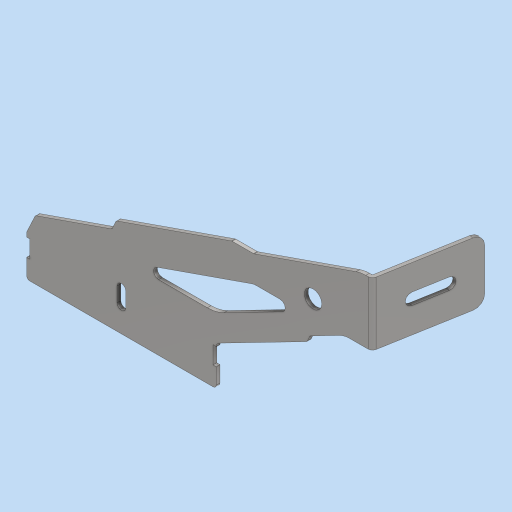
# Autodesk Inventor part: 0 零件
Saved by Autodesk Inventor 2023 (Build 270158000, 158)
## iProperties
Created: 2020-11-03
Part Number: 0 零件
Material: 不鏽鋼
Document SubType Name: Sheet Metal
Designer: p2013
Density: 8 g/cm^3
Appearance: SUS-2B
Sheet Metal Rule: 預設 mm (_M)
Flat Pattern Width: 8.37536 cm
Flat Pattern Length: 32.0542 cm
Flat Pattern Area: 268.466 cm^2
Sheet Metal Width: 83.754 mm
Sheet Metal Length: 320.542 mm
Sheet Metal Area: 26846.580 mm^2
Author: p2013
Autodesk Inventor part; units mm, degrees
ref_plane "YZ Plane" through (0, 0, 0) normal (1, 0, 0) x (0, 1, 0)
ref_plane "XZ Plane" through (0, 0, 0) normal (0, 1, 0) x (-1, 0, 0)
ref_plane "XY Plane" through (0, 0, 0) normal (0, 0, 1) x (1, 0, 0)
sketch "草圖1" plane through (0, 0, 0) normal (0, 0, 1) x (1, 0, 0)
  line L0 (0, 0) -> (-7.8042, 0) construction
  line L1 (0, 0) -> (0, -16.694) construction
  line L2 (0, 2) -> (0, 13)
  line L3 (234.1969, 118.5697) -> (234.1969, 75.5697)
  line L4 (130, 19.7875) -> (130, 13) construction
  line L5 (128, 0) -> (2, 0)
  line L6 (234.1969, 118.5697) -> (292.1969, 118.5697)
  line L7 (299.1969, 111.5697) -> (299.1969, 82.5697)
  line L8 (292.1969, 75.5697) -> (234.1969, 75.5697)
  line L9 (256.1969, 101.0697) -> (278.1969, 101.0697)
  arc A0 (278.1969, 93.0697) -> (278.1969, 101.0697) centre (278.1969, 97.0697) ccw
  line L10 (278.1969, 93.0697) -> (256.1969, 93.0697)
  arc A1 (256.1969, 101.0697) -> (256.1969, 93.0697) centre (256.1969, 97.0697) ccw
  line L11 (65, 14) -> (65, 14) construction
  line L12 (6.5315, 40.9329) -> (57.8672, 58.8322)
  line L13 (232.5836, 118.5697) -> (234.1969, 118.5697)
  line L14 (234.1969, 75.5697) -> (221.4643, 75.5697)
  line L15 (214.6027, 73.9083) -> (194.8909, 63.7682)
  arc A2 (299.1969, 111.5697) -> (292.1969, 118.5697) centre (292.1969, 111.5697) ccw
  arc A3 (292.1969, 75.5697) -> (299.1969, 82.5697) centre (292.1969, 82.5697) ccw
  line L16 (0, 25) -> (2.15, 25)
  line L17 (2.15, 25) -> (2.15, 13)
  line L18 (2.15, 13) -> (0, 13)
  line L19 (0, 13) -> (0, 25) construction
  line L20 (65, 0) -> (65, 27) construction
  line L21 (130, 25) -> (127.85, 25)
  line L22 (127.85, 25) -> (127.85, 13)
  line L23 (127.85, 13) -> (130, 13)
  line L24 (130, 13) -> (130, 19.7875) construction
  arc A4 (0, 2) -> (2, 0) centre (2, 2) ccw
  arc A5 (128, 0) -> (130, 2) centre (128, 2) ccw
  line L25 (0, 13) -> (0, 25) construction
  line L26 (0, 25) -> (0, 27.6675)
  line L27 (130, 19.7875) -> (130, 25) construction
  line L28 (130, 13) -> (130, 2)
  line L29 (123.9345, 45) -> (90.5004, 45)
  line L30 (157.566, 75) -> (173.8509, 75)
  line L31 (89.3481, 51.8049) -> (154.2737, 74.4425)
  line L32 (175.452, 68.3877) -> (135.3705, 47.769)
  arc A6 (175.452, 68.3877) -> (173.8509, 75) centre (173.8509, 71.5) ccw
  arc A7 (89.3481, 51.8049) -> (90.5004, 45) centre (90.5004, 48.5) ccw
  arc A8 (123.9345, 45) -> (135.3705, 47.769) centre (123.9345, 70) ccw
  arc A9 (157.566, 75) -> (154.2737, 74.4425) centre (157.566, 65) ccw
  line L33 (219.0826, 147.5779) -> (251.7371, 53.9233) construction
  arc A10 (232.5836, 118.5697) -> (225.9989, 117.4547) centre (232.5836, 98.5697) ccw
  arc A11 (221.4643, 75.5697) -> (214.6027, 73.9083) centre (221.4643, 60.5697) ccw
  line L34 (5.6659, 40.1505) -> (0.1405, 28.3014)
  line L35 (58.7328, 59.6146) -> (61.1461, 64.79)
  line L36 (62.0118, 65.5724) -> (140.4352, 92.9164)
  line L37 (140.9291, 93) -> (155.6079, 93)
  line L38 (131.899, 27.9903) -> (191.8622, 58.8365)
  line L39 (192.6867, 59.7276) -> (193.9617, 62.764)
  line L40 (194.2436, 63.4352) -> (119.2993, 24.8824) construction
  line L41 (156.1018, 93.0836) -> (225.9989, 117.4547)
  line L42 (58.4652, 59.0406) -> (155.8619, 93) construction
  arc A12 (194.8909, 63.7682) -> (193.9617, 62.764) centre (195.8058, 61.9897) ccw
  arc A13 (57.8672, 58.8322) -> (58.7328, 59.6146) centre (57.3734, 60.2485) ccw
  arc A14 (155.6079, 93) -> (156.1018, 93.0836) centre (155.6079, 94.5) ccw
  arc A15 (140.9291, 93) -> (140.4352, 92.9164) centre (140.9291, 91.5) ccw
  arc A16 (62.0118, 65.5724) -> (61.1461, 64.79) centre (62.5056, 64.1561) ccw
  arc A17 (191.8622, 58.8365) -> (192.6867, 59.7276) centre (191.0504, 60.4147) ccw
  circle A18 centre (196.4588, 86.5036) radius 6
  line L43 (130, 25) -> (130, 24.8779)
  arc A19 (131.899, 27.9903) -> (130, 24.8779) centre (133.5, 24.8779) ccw
  arc A20 (6.5315, 40.9329) -> (5.6659, 40.1505) centre (7.0253, 39.5165) ccw
  arc A21 (0.1405, 28.3014) -> (0, 27.6675) centre (1.5, 27.6675) ccw
  arc A22 (65, 24) -> (68, 27) centre (65, 27) ccw construction
  line L44 (62, 27) -> (62, 17)
  arc A23 (62, 17) -> (68, 17) centre (65, 17) ccw
  line L45 (68, 17) -> (68, 27)
  arc A24 (62, 27) -> (65, 24) centre (65, 27) ccw construction
  arc A25 (68, 27) -> (62, 27) centre (65, 27) ccw
  point P0 (130, 0)
  point P1 (299.1969, 118.5697)
  point P2 (299.1969, 75.5697)
  point P3 (0, 28)
  point P4 (130, 30.3871)
  point P5 (5.9335, 40.7244)
  point P6 (229.1969, 118.5697)
  point P7 (0, 10.2)
  point P8 (130, 28)
  point P9 (130, 10.2)
  point P10 (61.4138, 65.364)
  point P11 (140.6751, 93)
  point P12 (192.4366, 59.132)
  dimension "d0" = 130
  dimension "d2" = 43
  dimension "d3" = 65
  dimension "d4" = 8
  dimension "d5" = 30
  dimension "d7" = 18
  dimension "d14" = 14
  dimension "d17" = 21.5
  dimension "d21" = 28
  dimension "d23" = 5
  dimension "d24" = 7
  dimension "d33" = 8
  dimension "d39" = 12
  dimension "d41" = 13
  dimension "d42" = 2
  dimension "d46" = 17
  dimension "d47" = 13
  dimension "d49" = 3.5
  dimension "d50" = 3.5
  dimension "d51" = 25
  dimension "d52" = 10
  dimension "d57" = 4.7213
  dimension "d58" = 132.7034
  dimension "d60" = 19.222
  dimension "d61" = 20
  dimension "d62" = 15
  dimension "d65" = 118.5697
  dimension "d66" = 65
  dimension "d67" = 5
  dimension "d69" = 65
  dimension "d70" = 3
  dimension "d72" = 2
  dimension "d73" = 1.5
  dimension "d76" = 18
  dimension "d77" = 12
  dimension "d79" = 40
  dimension "d80" = 3.5
  dimension "d81" = 13.5
  dimension "d82" = 13.5
  dimension "d83" = 75
  dimension "d84" = 27.9903
  dimension "d85" = 45
  dimension "d86" = 55
  dimension "d87" = 1.5
  dimension "d91" = 10
  dimension "d93" = 6
  dimension "d94" = 17
  dimension "d95" = 125.7
  constraints: 94 end point, 54 tangent, 50 point on circle, 33 point on line, 26 centre point, 23 parallel, 9 horizontal, 8 perpendicular, 7 vertical, 6 equal radius, 5 symmetric about line, 3 vertical alignment, 2 coincident, 2 midpoint
  measures "d0" distance between parallel lines of L4 L2
  measures "d2" distance between parallel lines of L6 L8
  measures "d3" distance between parallel lines of L7 L3
  measures "d4" distance between parallel lines of L10 L9
  measures "d7" distance edge to line of A1 L3
  measures "d14" distance from line of L5 L11.start
  measures "d17" distance from line of L6 A0.centre
  measures "d21" distance of L0.start point (0, 28)
  measures "d23" distance of point (229.197, 118.57) L3.start
  measures "d24" radius of A2
  measures "d33" angle of L15 L12
  measures "d39" distance between parallel lines of L18 L16
  measures "d41" distance between parallel lines of L18 L5
  measures "d42" radius of A4
  measures "d46" distance between parallel lines of L12 L31
  measures "d47" distance between parallel lines of L15 L32
  measures "d49" radius of A6
  measures "d50" radius of A7
  measures "d51" radius of A8
  measures "d52" radius of A9
  measures "d57" distance from line of L3.start L33
  measures "d58" distance from line of point (130, 0) L33
  measures "d60" angle of L5 L12
  measures "d61" radius of A10
  measures "d62" radius of A11
  measures "d65" distance between parallel lines of L5 L6
  measures "d66" angle of L5 L34
  measures "d67" distance between parallel lines of L36 L12
  measures "d69" angle of L5 L35
  measures "d70" distance between parallel lines of L15 L38
  measures "d72" radius of A12
  measures "d73" radius of A13
  measures "d76" distance between parallel lines of L37 L30
  measures "d77" diameter of A18
  measures "d79" angle of L38 L39
  measures "d80" radius of A19
  measures "d81" distance edge to line of A18 L15
  measures "d82" distance edge to line of A18 L41
  measures "d83" distance between parallel lines of L5 L30
  measures "d84" distance from line of L38.start L5
  measures "d85" distance between parallel lines of L5 L29
  measures "d86" distance of point (5.933, 40.724) L12.end
  measures "d87" radius of A20
  measures "d91" distance of L20.end A23.centre
  measures "d93" distance between parallel lines of L45 L44
  measures "d94" distance from line of L5 A23.centre
  measures "d95" distance between parallel lines of L17 L22
extrude "擠出1" add sketch "草圖1" along normal blind 2.5
bend part "折彎零件1" radius 0.5 angle 80 line through (234.1969, 118.5697, 0) along (0, -1, 0) centre toward (0, 0, -1) moving side (1, 0, 0) both sides no
ref_plane "工作平面1" through (65, 2, 0) normal (-1, 0, 0) x (0, 0, 1)
